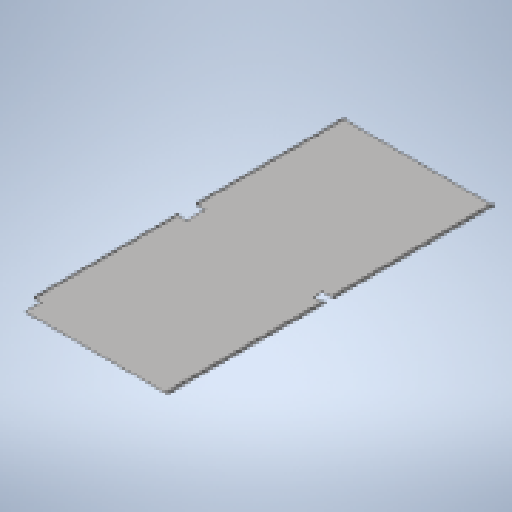
# Autodesk Inventor part: MSC 0101 sheet gills
Saved by Autodesk Inventor 2025 (Build 290162010, 162A)
## iProperties
Created: 2024-06-15
Part Number: MSC 0101 sheet gills
Material: Stainless Steel
Document SubType Name: Sheet Metal
Designer: pokla
Density: 8 g/cm^3
Sheet Metal Rule: Default_mm
Appearance: Default
Stock Number: МОО 0101 лист жабра
Mass: 7357.89 g
Surface Area: 36818.7 cm^2
Volume: 919.736 cm^3
Flat Pattern Width: 95.6524 cm
Flat Pattern Length: 200 cm
Flat Pattern Area: 19130.5 cm^2
Sheet Metal Width: 956,524 mm
Sheet Metal Length: 2000,000 mm
Sheet Metal Area: 1913047,787 mm^2
Author: pokla
Autodesk Inventor part; units mm, degrees
ref_plane "YZ Plane" through (0, 0, 0) normal (1, 0, 0) x (0, 1, 0)
ref_plane "XZ Plane" through (0, 0, 0) normal (0, 1, 0) x (-1, 0, 0)
ref_plane "XY Plane" through (0, 0, 0) normal (0, 0, 1) x (1, 0, 0)
sketch "Sketch6" plane through (0, 0, 0) normal (0, 1, 0) x (-1, 0, 0)
  line L0 (460, -1000) -> (-460, -1000)
  line L1 (-460, -1000) -> (-460, 1000)
  line L2 (-460, 1000) -> (460, 1000)
  line L3 (460, 1000) -> (460, -1000)
  line L4 (460, -1000) -> (-460, 1000) construction
  line L5 (-460, -1000) -> (460, 1000) construction
  point P0 (0, 0)
  dimension "d52" = 920
  dimension "d53" = 2000
  measures "d52" distance of L1.end L2.end
  measures "d53" distance of L0.end L1.end
extrude "Plate2" add sketch "Sketch6" along normal blind 0.5
sketch "Sketch10" plane through (-459.5, 0, 1000) normal (-1, 0, 0) x (0, -1, 0)
  line L0 (0, -2000) -> (0, 0)
  line L1 (0, 0) -> (-10, 0)
  line L2 (-10, 0) -> (-10, -2000)
  line L3 (-10, -2000) -> (0, -2000)
  constraints: 6 end point, 1 horizontal, 1 perpendicular, 1 vertical
edge flange "Flange1" height 10 angle 90 thickness 0.5 bend radius 0.5 thickness toward (-1, 0, 0) relief straight relief width 0.5 relief depth 0.25 corner gap 0.5 corner form 0 edges at (-460, 0.5, 0) (460, 0.5, 0) wall of the first edge with corners at (-459.5, 0, -1000) (-459.5, 0, 1000) (-459.5, 10, 1000) (-459.5, 10, -1000)
bend "Bend2"
corner "Corner2"
sketch "Sketch11" plane through (460, 9.5, -1000) normal (0, 1, 0) x (-1, 0, 0)
  line L0 (0, 2000) -> (0, 0)
  line L1 (0, 0) -> (10, 0)
  line L2 (10, 0) -> (10, 2000)
  line L3 (10, 2000) -> (0, 2000)
  constraints: 6 end point, 1 horizontal, 1 perpendicular, 1 vertical
edge flange "Flange2" height 10 angle 90 thickness 0.5 bend radius 0.5 thickness toward (0, 1, 0) relief straight relief width 0.5 relief depth 0.25 corner gap 0.5 corner form 0 edges at (459.5, 10, 0) (-459.5, 10, 0) wall of the first edge with corners at (460, 9.5, 1000) (460, 9.5, -1000) (450, 9.5, -1000) (450, 9.5, 1000)
bend "Bend3"
corner "Corner3"
sketch "Sketch12" plane through (0, 0, 0) normal (0, -1, 0) x (1, 0, 0)
  line L0 (460, -1000) -> (460, 1000) projected
  line L1 (460, 1000) -> (460, -1000) projected
  line L2 (-460, -1000) -> (-460, 1000) projected
  line L3 (-460, 1000) -> (-416.61, 1000)
  line L4 (-416.61, 1000) -> (-416.61, 899.713)
  line L5 (-416.61, 899.713) -> (-460, 899.713)
  line L6 (-460, 899.713) -> (-460, 1000)
  line L7 (-460, 20.3845) -> (-405.6681, 20.3845)
  line L8 (-405.6681, 20.3845) -> (-405.6681, -94.3031)
  line L9 (-405.6681, -94.3031) -> (-460, -94.3031)
  line L10 (-460, -94.3031) -> (-460, 20.3845)
  line L11 (460, 35.0533) -> (389.3937, 35.0533)
  line L12 (389.3937, 35.0533) -> (389.3937, -18.4335)
  line L13 (389.3937, -18.4335) -> (460, -18.4335)
  line L14 (460, -18.4335) -> (460, 35.0533)
  point P0 (0, 0)
  constraints: 24 end point, 6 parallel, 3 horizontal, 3 perpendicular, 2 point on line
extrude "Extrusion3" cut sketch "Sketch12" along normal through all both and the other way through all
equation "\"d54\" = Thickness"
equation "\"d74\" = BendReliefWidth"
equation "\"d75\" = BendReliefDepth"
equation "\"d76\" = MinimumRemnant"
equation "\"d77\" = TransitionRadius"
equation "\"d80\" = BendRadius"
equation "\"d81\" = CornerReliefSize"
equation "\"d82\" = GapSize"
equation "\"d83\" = JacobiRadiusSize"
equation "\"d84\" = BendReliefWidth"
equation "\"d85\" = BendReliefDepth"
equation "\"d86\" = MinimumRemnant"
equation "\"d87\" = TransitionRadius"
equation "\"d90\" = BendRadius"
equation "\"d91\" = CornerReliefSize"
equation "\"d92\" = GapSize"
equation "\"d93\" = JacobiRadiusSize"
equation "\"BendRadius\" = Thickness"
equation "\"BendReliefWidth\" = Thickness"
equation "\"BendReliefDepth\" = 0.5 * Thickness"
equation "\"CornerReliefSize\" = 4 * Thickness"
equation "\"MinimumRemnant\" = 2 * Thickness"
equation "\"TransitionRadius\" = BendRadius"
equation "\"JacobiRadiusSize\" = BendRadius"
equation "\"GapSize\" = Thickness"
equation "\"Thickness\" = 0.5"
body "Solid2"
